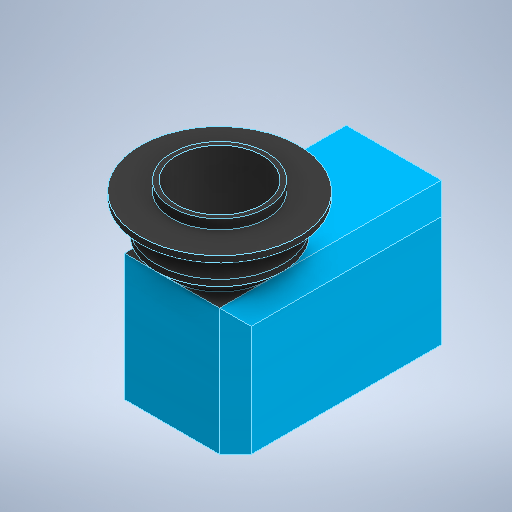
# Autodesk Inventor part: part
Saved by Autodesk Inventor 2025 (Build 290162000, 162)
## iProperties
Created: 2024-09-26
Part Number: part
Material: ABS Plastic
Document SubType Name: Modeling
Designer: DMIADX
Density: 1.06 g/cm^3
Appearance: Sky Blue Medium
Author: DMIADX
Autodesk Inventor part; units mm, degrees
sketch "Sketch1" plane through (0, 0, 0) normal (0, 1, 0) x (-1, 0, 0)
  line L0 (-20, 35) -> (20, 35)
  line L1 (20, 35) -> (20, -35)
  line L2 (20, -35) -> (-20, -35)
  line L3 (-20, -35) -> (-20, 35)
  line L4 (-20, 35) -> (20, -35) construction
  line L5 (20, 35) -> (-20, -35) construction
  line L6 (-17.5, 35) -> (17.5, 35)
  line L7 (17.5, 35) -> (17.5, -35)
  line L8 (17.5, -35) -> (-17.5, -35)
  line L9 (-17.5, -35) -> (-17.5, 35)
  line L10 (-17.5, 35) -> (17.5, -35) construction
  line L11 (17.5, 35) -> (-17.5, -35) construction
  line L12 (-20, 20) -> (20, 20)
  line L13 (20, 20) -> (20, -20)
  line L14 (20, -20) -> (-20, -20)
  line L15 (-20, -20) -> (-20, 20)
  line L16 (-20, 20) -> (20, -20) construction
  line L17 (20, 20) -> (-20, -20) construction
  point P0 (0, 0)
  dimension "d0" = 40
  dimension "d1" = 70
  dimension "d2" = 40
  dimension "d3" = 35
  constraints: 36 end point, 6 midpoint, 6 parallel, 3 horizontal, 3 perpendicular, 2 point on line
  measures "d0" distance between parallel lines of L3 L1
  measures "d1" distance between parallel lines of L0 L2
  measures "d2" distance between parallel lines of L12 L14
  measures "d3" distance between parallel lines of L9 L7
extrude "Extrusion1" add sketch "Sketch1" along normal blind 40
chamfer "Chamfer1" distance 5 angle 45 4 edges at (20, 20, 35) (-20, 20, 35) (-20, 20, -35) (20, 20, -35)
ref_plane "Work Plane1" through (0, 10, 0) normal (0, -1, 0) x (1, 0, 0)
chamfer "Chamfer2" distance 5 angle 45 2 edges at (20, 40, 0) (-20, 40, 0)
ref_plane "Work Plane3" through (0, 0, 30) normal (1, 0, 0) x (0, 0, -1)
sketch "Sketch5" plane through (0, 0, 30) normal (1, 0, 0) x (0, 0, -1)
  point P0 (30, 0)
sketch "Sketch6" plane through (0, 10, 0) normal (0, -1, 0) x (1, 0, 0)
  point P0 (0, 0)
sketch "Sketch7" plane through (0, 0, 30) normal (1, 0, 0) x (0, 0, -1)
  line L0 (-5, 40) -> (65, 40) projected
  line L1 (10, 40) -> (10, 60)
  line L2 (-5, 0) -> (-5, 40) projected
  line L3 (-5, 40) -> (-10, 45)
  line L4 (-10, 45) -> (-10, 47)
  line L5 (-10, 47) -> (-5, 52)
  line L6 (-5, 52) -> (-5, 55)
  line L7 (-5, 55) -> (-15, 55)
  line L8 (-5, 57) -> (-5, 60)
  line L9 (-5, 60) -> (10, 60)
  line L10 (-15, 57) -> (-5, 57)
  line L11 (-15, 55) -> (-15, 57)
  point P0 (30, 0)
  point P1 (-10, 46)
  point P2 (-22, 56)
  point P3 (-5, 58.5)
  point P4 (-5, 53.5)
  point P5 (-15, 56)
  point P6 (-10, 57)
  dimension "d34" = 20
  dimension "d35" = 15
  dimension "d37" = 12
  dimension "d39" = 5
  dimension "d40" = 2
  dimension "d42" = 40
  dimension "d43" = 64
  dimension "d44" = 30
  dimension "d45" = 30
  dimension "d46" = 50
  dimension "d47" = 2
  dimension "d48" = 3
  constraints: 20 end point, 5 midpoint, 4 perpendicular, 1 horizontal, 1 parallel, 1 point on line, 1 vertical
  measures "d34" distance of L1.start L1.end
  measures "d35" distance between parallel lines of L2 L1
  measures "d37" distance of L5.end L0.start
  measures "d39" distance from line of L0 L3.end
  measures "d40" distance of L3.end L4.end
  measures "d42" diameter of point (-10, 46) L1
  measures "d43" diameter of point (-22, 56) L1
  measures "d44" diameter of point (-5, 58.5) L1
  measures "d45" diameter of point (-5, 53.5) L1
  measures "d46" diameter of point (-15, 56) L1
  measures "d47" distance from line of L7 point (-10, 57)
  measures "d48" distance between parallel lines of L9 L10
revolve "Revolution2" add sketch "Sketch7" angle 360 about axis through (0, 40, 20) along (0, 1, 0)
sketch "Sketch8" plane through (0, 60, 20) normal (0, 1, 0) x (1, 0, 0)
  point P0 (0, 20)
  point P1 (0, 0)
hole "Hole1" at (0, 60, 20) direction (0, -1, 0) diameter 27 depth 20
sketch "Sketch9" plane through (-20, 0, -30) normal (-1, 0, 0) x (0, 0, 1)
  circle A0 centre (50, 27.008) radius 2.4494
  point P0 (30, 0)
  constraints: 1 centre point
extrude "Extrusion4" add sketch "Sketch9" along normal blind 5
fillet "Fillet1" radius 1 1 edges at (-25, 27.008, 17.5506)
sketch "Sketch10" plane through (-20, 0, -30) normal (-1, 0, 0) x (0, 0, 1)
  line L0 (33, 29) -> (45, 29)
  line L1 (45, 29) -> (45, 19)
  line L2 (45, 19) -> (33, 19)
  line L3 (33, 19) -> (33, 29)
  line L4 (33, 26) -> (37, 26)
  line L5 (39, 24) -> (39, 19)
  line L6 (60, 35) -> (60, 0) projected
  line L7 (0, 35) -> (60, 35) projected
  line L8 (37, 26) -> (39, 24)
  line L9 (38.2426, 29) -> (45, 22.2426)
  line L10 (42, 30.25) -> (42, 15.4606)
  line L11 (38, 22) -> (48.4916, 22)
  line L12 (44, 22) -> (44, 19)
  point P0 (30, 0)
  point P1 (39, 26)
  point P2 (39, 21.5)
  point P3 (39, 29)
  point P4 (45, 24)
  point P5 (38, 25)
  point P6 (45, 22)
  point P7 (42, 22)
  point P8 (42, 25.2426)
  dimension "d60" = 6
  dimension "d61" = 10
  dimension "d62" = 12
  dimension "d63" = 15
  dimension "d64" = 16
  dimension "d65" = 3
  dimension "d66" = 2
  dimension "d67" = 2
  dimension "d68" = 3
  dimension "d69" = 3
  dimension "d70" = 3
  dimension "d73" = 1
  constraints: 22 end point, 7 point on line, 5 midpoint, 3 horizontal, 3 parallel, 3 perpendicular, 1 vertical
  measures "d60" distance from line of L1 point (39, 21.5)
  measures "d61" distance from line of point (39, 29) L2
  measures "d62" distance between parallel lines of L3 L1
  measures "d63" distance from line of L6 point (45, 24)
  measures "d64" distance between parallel lines of L7 L2
  measures "d65" distance between parallel lines of L0 L4
  measures "d66" distance of L4.end point (39, 26)
  measures "d67" distance of L5.start point (39, 26)
  measures "d68" distance between parallel lines of L5 L10
  measures "d69" distance from line of point (38, 25) L9
  measures "d70" distance between parallel lines of L2 L11
  measures "d73" distance between parallel lines of L1 L12
extrude "Extrusion5" add sketch "Sketch10" along normal blind 4 contours L0 L9 L10 L11 L5 L8 L4 L3 | L11 L12 L2 L10 | L10 L2 L5 L11 | L1 L2 L12 L11
extrude "Extrusion6" cut sketch "Sketch10" along normal blind 3 contours L0 L9 L10 L11 L5 L8 L4 L3 | L11 L12 L2 L10 | L10 L2 L5 L11
sketch "Sketch11" plane through (-24, 0, -30) normal (-1, 0, 0) x (0, 0, 1)
  line L0 (33, 29) -> (33, 26) projected
  line L1 (38.2426, 29) -> (33, 29) projected
  line L2 (34, 26) -> (34, 29)
  line L3 (33, 29) -> (33, 26)
  line L4 (33, 26) -> (33, 25)
  line L5 (33, 25) -> (34, 25)
  line L6 (34, 25) -> (34, 26)
  line L7 (33, 30) -> (34, 30)
  line L8 (33, 29) -> (33, 30)
  line L9 (34, 30) -> (34, 29)
  point P0 (30, 0)
  point P1 (33.5, 25)
  dimension "d76" = 1
  constraints: 16 end point, 2 perpendicular, 1 midpoint, 1 parallel, 1 point on line, 1 vertical
  measures "d76" distance between parallel lines of L0 L2
extrude "Extrusion7" add sketch "Sketch11" along normal blind 8
sketch "Sketch12" plane through (-24, 25, 4) normal (0, 0, 1) x (1, 0, 0)
  line L0 (-8.9741, 1.75) -> (-1, 1.75)
  line L1 (-1, 1.75) -> (-1, 3.25)
  line L2 (-1, 3.25) -> (-8.9741, 3.25)
  line L3 (-8.9741, 3.25) -> (-8.9741, 1.75)
  line L4 (0, 0) -> (-8, 0) projected
  line L5 (-8, 0) -> (-8, 5) projected
  point P0 (24, -25)
  point P1 (-8, 3.25)
  point P2 (-8, 1.75)
  dimension "d80" = 1.5
  dimension "d81" = 1.75
  dimension "d82" = 7
  constraints: 8 end point, 2 parallel, 1 horizontal, 1 perpendicular
  measures "d80" distance between parallel lines of L2 L0
  measures "d81" distance between parallel lines of L4 L0
  measures "d82" distance between parallel lines of L5 L1
extrude "Extrusion8" cut sketch "Sketch12" against normal blind 8 contours L5 L2 L1 L0
fillet "Fillet2" radius 0.5 6 edges at (-32, 25, 3.5) (-32, 30, 3.5) (-32, 26.75, 3.5) (-32, 28.25, 3.5) (-25, 28.25, 3.5) (-25, 26.75, 3.5)
sketch "Sketch13" plane through (-20, 0, -30) normal (-1, 0, 0) x (0, 0, 1)
  point P0 (30, 0)
sketch "Sketch14" plane through (-20, 0, -30) normal (-1, 0, 0) x (0, 0, 1)
  line L0 (0, 35) -> (0, 0) projected
  line L1 (60, 0) -> (60, 35) projected
  point P0 (30, 0)
sketch "Sketch15" plane through (-24, 0, -30) normal (-1, 0, 0) x (0, 0, 1)
  point P0 (30, 0)
ref_plane "Work Plane4" through (-24, 20.5, 15) normal (0, -1, 0) x (1, 0, 0)
mirror "Mirror2" about plane through (-24, 20.5, 15) normal (0, -1, 0) of "Extrusion5", "Extrusion6", "Extrusion7", "Extrusion8"
equation "\"d67\" = d66"
body "Solid1"
